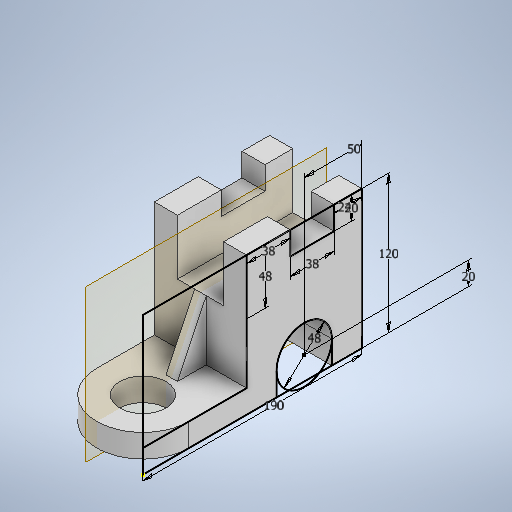
# Autodesk Inventor part: 2
Saved by Autodesk Inventor 2025.2 (Build 292293000, 293)
## iProperties
Created: 2024-12-04
Part Number: 2
Material: Generic
Document SubType Name: Modeling
Designer: hongquan
Density: 1 g/cm^3
Appearance: Default
Author: hongquan
Autodesk Inventor part; units mm, degrees
ref_plane "XZ Plane" through (0, 0, 0) normal (0, 1, 0) x (-1, 0, 0)
ref_plane "XY Plane" through (0, 0, 0) normal (0, 0, 1) x (1, 0, 0)
sketch "Sketch1" plane through (0, 0, 0) normal (1, 0, 0) x (0, 1, 0)
  point P0 (0, 0)
sketch "Sketch2" plane through (0, 0, 0) normal (1, 0, 0) x (0, 1, 0)
  line L0 (0, 0) -> (120, 0)
  line L1 (120, 0) -> (120, -190)
  line L2 (120, -190) -> (0, -190)
  line L3 (0, -190) -> (0, 0)
  circle A0 centre (20, -140) radius 24
  line L4 (20, -164) -> (0, -164)
  line L5 (20, -116) -> (0, -116)
  line L6 (120, -190) -> (120, -166)
  line L7 (120, -166) -> (100, -166)
  line L8 (100, -166) -> (100, -128)
  line L9 (100, -128) -> (120, -128)
  line L10 (120, -128) -> (120, -90)
  line L11 (120, -90) -> (72, -90)
  line L12 (72, -90) -> (20, -90)
  line L13 (20, -90) -> (20, 0)
  line L14 (20, 0) -> (0, 0)
  line L15 (120, 0) -> (20, 0)
  point P0 (0, -126.7335)
  point P1 (0, -153.2665)
  dimension "d0" = 190
  dimension "d1" = 120
  dimension "d4" = 48
  dimension "d5" = 20
  dimension "d6" = 50
  dimension "d7" = 24
  dimension "d8" = 20
  dimension "d9" = 38
  dimension "d10" = 38
  dimension "d11" = 48
  constraints: 32 end point, 7 perpendicular, 6 point on line, 4 horizontal, 2 parallel, 2 point on circle, 2 vertical, 1 centre point, 1 collinear, 1 tangent
  measures "d0" distance of L2.end L0.start
  measures "d1" distance of L2.end L1.end
  measures "d4" diameter of A0
  measures "d5" distance from line of L3 A0.centre
  measures "d6" distance from line of L2 A0.centre
  measures "d7" distance of L1.end L6.end
  measures "d8" distance of L6.end L7.end
  measures "d9" distance of L7.end L8.end
  measures "d10" distance of L9.end L10.end
  measures "d11" distance of L10.end L11.end
extrude "Extrusion1" add sketch "Sketch2" against normal blind 80 contours L0 L13 L12 L11 L1 L9 L8 L7 L2 L3 L4 A0 L5 | L0 L1 L11 L12 L13 | L5 A0 L3 | A0 L3 | A0 L4 L3 | L1 L7 L8 L9 picked at (15.1537, -135.0371)
extrude "Extrusion2" cut sketch "Sketch2" against normal blind 80 contours L0 L1 L11 L12 L13 | A0 L3 | L1 L7 L8 L9 picked at (15.1537, -135.0371)
extrude "Extrusion3" cut sketch "Sketch2" against normal blind 80 contours L5 A0 L3 | A0 L4 L3
sketch "Sketch3" plane through (-80, 20, -90) normal (0, 1, 0) x (1, 0, 0)
  line L0 (80, -90) -> (0, -90) projected
  line L1 (40, -90) -> (40, 100)
  line L2 (80, 100) -> (0, 100) projected
  circle A0 centre (40, -50) radius 20
  circle A1 centre (40, -50) radius 40
  line L3 (80, -90) -> (0, -90) projected
  line L4 (0, -90) -> (0, 0) projected
  line L5 (0, -90) -> (0, 100)
  line L6 (0, -90) -> (80, -90)
  line L7 (80, 74) -> (80, 100) projected
  line L8 (80, -90) -> (80, 100)
  point P0 (80, -50)
  point P1 (0, -50)
  dimension "d16" = 40
  dimension "d17" = 80
  dimension "d18" = 40
  constraints: 8 end point, 3 midpoint, 2 centre point, 2 perpendicular, 1 coincident, 1 collinear, 1 point on line
  measures "d16" diameter of A0
  measures "d17" diameter of A1
  measures "d18" distance of A1.centre point (40, -90)
extrude "Extrusion4" cut sketch "Sketch3" against normal blind 80 contours L0 A1 L8 | L0 L4 A1 | A0 L1 | L1 A0
sketch "Sketch4" plane through (-80, 120, -90) normal (0, 0, 1) x (1, 0, 0)
  line L0 (0, 0) -> (0, -120) projected
  line L1 (80, 0) -> (80, -100) projected
  line L2 (0, 0) -> (80, 0)
  line L3 (80, 0) -> (80, -120)
  line L4 (0, -120) -> (80, -120) projected
  line L5 (80, -120) -> (0, -120)
  line L6 (0, -120) -> (0, 0)
  line L7 (80, 0) -> (0, 0) projected
  line L8 (40, 0) -> (40, -120)
  line L9 (0, 0) -> (0, -48)
  line L10 (0, 0) -> (20, 0)
  line L11 (20, 0) -> (20, -48)
  line L12 (20, -48) -> (60, -48)
  line L13 (60, -48) -> (60, 0)
  dimension "d21" = 48
  dimension "d22" = 20
  dimension "d23" = 40
  dimension "d24" = 48
  constraints: 20 end point, 6 perpendicular, 3 point on line, 2 midpoint, 1 horizontal
  measures "d21" distance of L0.start L9.end
  measures "d22" distance of L0.start L10.end
  measures "d23" distance of L11.end L12.end
  measures "d24" distance of L12.end L13.end
extrude "Extrusion5" cut sketch "Sketch4" against normal blind 100 contours L2 L8 L12 L11 | L2 L13 L12 L8
ref_plane "Work Plane1" through (-40, 72, -90) normal (1, 0, 0) x (0, 1, 0)
sketch "Sketch5" plane through (-40, 72, -90) normal (1, 0, 0) x (0, 1, 0)
  line L0 (0, 0) -> (0, -100) projected
  line L1 (0, 0) -> (0, 25)
  line L2 (0, 25) -> (-52, 25)
  line L3 (0, 0) -> (-52, 25)
  line L4 (-52, 50) -> (-52, 0) projected
  line L5 (0, 0) -> (-52, 0)
  line L6 (-52, 0) -> (-52, 25)
  point P0 (-72, 90)
  dimension "d27" = 25
  dimension "d28" = 52
  constraints: 10 end point, 2 perpendicular, 1 vertical
  measures "d27" distance of L0.start L1.end
  measures "d28" distance of L1.end L2.end
extrude "Extrusion6" add sketch "Sketch5" along normal mid plane 10 contours L5 L4 L3
body "Solid1"
